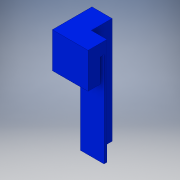
# Autodesk Inventor part: 8GrootTelescope
Saved by Autodesk Inventor 2018.3 (Build 223284000, 284)
## iProperties
Created: 2020-01-28
Part Number: 8GrootTelescope
Material: Generic
Document SubType Name: Modeling
Designer: 22perngrac
Density: 1 g/cm^3
Appearance: Default
Mass: 7.33252 g
Surface Area: 50.4971 cm^2
Volume: 7.33252 cm^3
Author: 22perngrac
Autodesk Inventor part; units mm, degrees
ref_plane "YZ Plane" through (0, 0, 0) normal (1, 0, 0) x (0, 1, 0)
ref_plane "XZ Plane" through (0, 0, 0) normal (0, 1, 0) x (-1, 0, 0)
ref_plane "XY Plane" through (0, 0, 0) normal (0, 0, 1) x (1, 0, 0)
sketch "Sketch1" plane through (0, 0, 0) normal (0, 1, 0) x (-1, 0, 0)
  line L0 (0, 0) -> (-12.7, 0)
  line L1 (-12.7, 0) -> (-12.7, -1.5875)
  line L2 (-12.7, -1.5875) -> (0, -1.5875)
  line L3 (0, -1.5875) -> (0, 0)
  line L4 (0, 0) -> (-4.318, 0)
  line L5 (-4.318, 0) -> (-4.318, -12.7)
  line L6 (-4.318, -12.7) -> (0, -12.7)
  line L7 (0, -12.7) -> (0, 0)
  dimension "d0" = 4.318
  dimension "d1" = 12.7
  dimension "d2" = 12.7
  dimension "d33" = 1.5875
  constraints: 16 end point, 4 parallel, 2 horizontal, 2 perpendicular
  measures "d0" distance of L5.end L6.end
  measures "d1" distance of L0.start L0.end
  measures "d2" distance of L6.end L0.start
  measures "d33" distance of L0.end L1.end
extrude "Extrusion1" add sketch "Sketch1" along normal blind 50.8
sketch "Sketch2" plane through (0, 50.8, 0) normal (0, 1, 0) x (1, 0, 0)
  line L0 (12.7, 0) -> (12.7, 1.5875) projected
  line L1 (12.7, 1.5875) -> (-4.064, 1.5875)
  line L2 (-4.064, 1.5875) -> (-4.064, -8.5725)
  line L3 (-4.064, -8.5725) -> (12.7, -8.5725)
  line L4 (12.7, -8.5725) -> (12.7, 1.5875)
  line L5 (4.318, 12.7) -> (-4.064, 12.7)
  line L6 (-4.064, 12.7) -> (-4.064, -8.5725)
  line L7 (-4.064, -8.5725) -> (4.318, -8.5725)
  line L8 (4.318, -8.5725) -> (4.318, 12.7)
  dimension "d26" = 10.16
  dimension "d28" = 16.764
  constraints: 16 end point, 4 parallel, 2 horizontal, 2 perpendicular
  measures "d26" distance of L3.end L0.end
  measures "d28" distance of L2.end L3.end
extrude "Extrusion2" add sketch "Sketch2" along normal blind 6.35
sketch "Sketch5" plane through (0, 50.8, 0) normal (0, -1, 0) x (1, 0, 0)
  line L0 (12.7, 8.5725) -> (12.7, 0) projected
  line L1 (-4.064, -12.7) -> (-4.064, 8.5725) projected
  line L2 (12.7, 8.5725) -> (-4.064, 8.5725)
  line L3 (-4.064, 8.5725) -> (-4.064, 2.1082)
  line L4 (-4.064, 2.1082) -> (12.7, 2.1082)
  line L5 (12.7, 2.1082) -> (12.7, 8.5725)
  line L6 (0, -12.7) -> (-4.064, -12.7) projected
  line L7 (-4.064, 8.5725) -> (-2.1082, 8.5725)
  line L8 (-2.1082, 8.5725) -> (-2.1082, -12.7)
  line L9 (-2.1082, -12.7) -> (-4.064, -12.7)
  line L10 (-4.064, -12.7) -> (-4.064, 8.5725)
  line L11 (0, -12.7) -> (0, 0) projected
  line L12 (0, 0) -> (12.7, 0) projected
  dimension "d29" = 2.1082
  dimension "d30" = 2.1082
  constraints: 16 end point, 4 parallel, 2 horizontal, 2 perpendicular, 2 point on line
  measures "d29" distance between parallel lines of L11 L8
  measures "d30" distance between parallel lines of L12 L4
extrude "Extrusion4" add sketch "Sketch5" along normal blind 12.7 contours L0 L4 L8 L2 | L8 L4 L1 L2 | L8 L6 L1 L4
sketch "Sketch7" plane through (-4.064, 57.15, -12.7) normal (-1, 0, 0) x (0, 0, 1)
  line L0 (11.1125, 0) -> (11.1125, -57.15) projected
  line L1 (0, -57.15) -> (0, 0) projected
  line L2 (11.1125, 0) -> (0, 0) projected
  line L3 (0, -19.05) -> (14.8082, -19.05) projected
  line L4 (0, -6.35) -> (12.7, -6.35) projected
  point P0 (12.7, -57.15)
  point P1 (5.5562, -12.7)
  dimension "d47" = 11.1125
  dimension "d49" = 5.5563
  dimension "d58" = 12.7
  dimension "d59" = 6.35
  measures "d47" distance between parallel lines of L0 L1
  measures "d49" distance from line of point (5.556, -12.7) L1
  measures "d58" distance between parallel lines of L4 L3
  measures "d59" distance from line of L4 point (5.556, -12.7)
hole "Hole2" at (-4.064, 44.45, -7.1438) direction (1, 0, 0) diameter 5.1562 depth 1.5875 tip angle 118
sketch "Sketch8" plane through (-4.064, 57.15, -12.7) normal (-1, 0, 0) x (0, 0, 1)
  circle A0 centre (5.5562, -12.7) radius 2.5781 projected
  circle A1 centre (5.5562, -12.7) radius 2.5781 projected
  line L0 (21.2725, 0) -> (21.2725, -19.05) projected
  line L1 (0, 0) -> (21.2725, 0) projected
  line L2 (0, -19.05) -> (0, 0) projected
  line L3 (21.2725, -19.05) -> (0, -19.05) projected
  point P0 (12.7, -57.15)
extrude "Extrusion5" add sketch "Sketch8" along normal blind 2.413
sketch "Sketch9" plane through (-2.1082, 50.8, 2.1082) normal (1, 0, 0) x (0, 0, -1)
  circle A0 centre (9.2519, -6.35) radius 2.5781 projected
  line L0 (14.8082, -12.7) -> (-6.4643, -12.7) projected
  line L1 (6.6738, -6.35) -> (11.83, -6.35)
  line L2 (11.83, -6.35) -> (11.83, -12.7)
  line L3 (11.83, -12.7) -> (6.6738, -12.7)
  line L4 (6.6738, -12.7) -> (6.6738, -6.35)
  point P0 (2.1082, -50.8)
  dimension "d62" = 5.1562
  constraints: 8 end point, 2 parallel, 2 point on circle, 1 horizontal, 1 perpendicular, 1 point on line
  measures "d62" distance of L1.start L1.end
extrude "Extrusion6" cut sketch "Sketch9" against normal blind 1.5875
equation "\"d29\" = d30"
equation "\"d49\" = 0.5 * d47"
equation "\"d59\" = 0.5 * d58"
body "Solid1"
